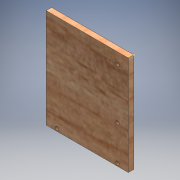
# Autodesk Inventor part: SideSupport
Saved by Autodesk Inventor 2016 (Build 200138000, 138)
## iProperties
Created: 2016-04-01
Part Number: SideSupport
Material: Wood (Birch)
Document SubType Name: Modeling
Designer: mkepler
Mass: 4.26525 g
Surface Area: 57.82 cm^2
Volume: 7.755 cm^3
Density: 0.55 g/cm^3
Appearance: Birch - Natural Polished
Author: mkepler
Autodesk Inventor part; units mm, degrees
ref_plane "YZ Plane" through (0, 0, 0) normal (1, 0, 0) x (0, 1, 0)
ref_plane "XZ Plane" through (0, 0, 0) normal (0, 1, 0) x (-1, 0, 0)
ref_plane "XY Plane" through (0, 0, 0) normal (0, 0, 1) x (1, 0, 0)
sketch "Sketch1" plane through (0, 0, 0) normal (0, 1, 0) x (-1, 0, 0)
  line L0 (0, 0) -> (45.5, 0)
  line L1 (45.5, 0) -> (45.5, -55)
  line L2 (45.5, -55) -> (0, -55)
  line L3 (0, -55) -> (0, 0)
  dimension "d0" = 45.5
  dimension "d1" = 55
  constraints: 8 end point, 2 parallel, 1 horizontal, 1 perpendicular
  measures "d0" distance of L1.end L2.end
  measures "d1" distance of L0.end L1.end
extrude "Extrusion1" add sketch "Sketch1" along normal blind 3
sketch "Sketch2" plane through (0, 3, 0) normal (0, 1, 0) x (1, 0, 0)
  line L0 (-45.5, 55) -> (-45.5, 0) projected
  line L1 (-45.5, 40) -> (0, 40)
  line L2 (0, 0) -> (0, 55) projected
  line L3 (0, 55) -> (-45.5, 55) projected
  circle A0 centre (-6, 34) radius 1
  circle A1 centre (-6, 6) radius 1
  line L4 (-45.5, 0) -> (0, 0) projected
  line L5 (0, 55) -> (-45.5, 55)
  line L6 (-45.5, 55) -> (-45.5, 52)
  line L7 (-45.5, 52) -> (0, 52)
  line L8 (0, 52) -> (0, 55)
  circle A2 centre (-6, 53.5) radius 0.5
  line L9 (-22.75, 55) -> (-22.75, 53.5)
  circle A3 centre (-39.5, 53.5) radius 0.5
  dimension "d4" = 15
  dimension "d5" = 2
  dimension "d6" = 6
  dimension "d7" = 6
  dimension "d8" = 2
  dimension "d9" = 6
  dimension "d10" = 6
  dimension "d18" = 3
  dimension "d19" = 1
  dimension "d20" = 6
  constraints: 12 end point, 4 centre point, 3 point on line, 2 horizontal, 2 parallel, 1 midpoint, 1 perpendicular, 1 symmetric about line, 1 vertical, 1 other
  measures "d4" distance between parallel lines of L3 L1
  measures "d5" diameter of A0
  measures "d6" distance from line of L1 A0.centre
  measures "d7" distance from line of L2 A0.centre
  measures "d8" diameter of A1
  measures "d9" distance from line of L2 A1.centre
  measures "d10" distance from line of L4 A1.centre
  measures "d18" distance of L6.end L5.end
  measures "d19" diameter of A2
  measures "d20" distance from line of L8 A2.centre
hole "Hole1" at (-6, 3, -6) at (-6, 3, -34) at (-6, 3, -53.5) at (-39.5, 3, -53.5) direction (0, -1, 0) diameter 2 end through all
sketch "Sketch3" plane through (0, 3, 0) normal (0, 1, 0) x (1, 0, 0)
  point P0 (0, 0)
body "Solid1"
